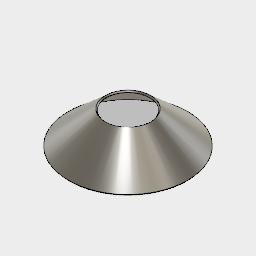
top_roof v3 (Autodesk Fusion 360 design; units mm, degrees)
Autodesk Fusion 360 part; units mm, degrees
sketch "スケッチ1" plane through (0, 0, 0) normal (0, 0, 1) x (1, 0, 0)
  line L0 (0, 0) -> (0, 35)
  line L1 (0, 35) -> (30, 35)
  line L2 (0, 0) -> (70, 0)
  line L3 (30, 35) -> (70, 0)
  line L4 (70, 0) -> (132.0268, -54.2735)
  line L5 (0, 0) -> (0, -10)
  line L6 (0, -10) -> (81.4286, -10)
  line L7 (30, 35) -> (81.4286, -10)
  line L8 (81.4286, -10) -> (83.0748, -8.1186)
  line L9 (83.0748, -8.1186) -> (31.6463, 36.8814)
  line L10 (31.6463, 36.8814) -> (30, 35)
  dimension "d1" = 35
  dimension "d2" = 30
  dimension "d3" = 70
  dimension "d4" = 10
  dimension "d5" = 2.5
  measures "d1" distance of L0.start L0.end
  measures "d2" distance of L0.end L1.end
  measures "d3" distance of L0.start L2.end
  measures "d4" distance of L0.start L5.end
  measures "d5" distance of L1.end L9.end
revolve "回転1" add sketch "スケッチ1" angle 360 about axis through (0, 0, 0) along (0, 1, 0) contours L3 L4 L7 L8 L9 L10
